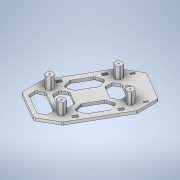
# Autodesk Inventor part: top_body
Saved by Autodesk Inventor 2022 (Build 260153000, 153)
## iProperties
Created: 2022-01-21
Part Number: top_body
Material: Generic
Document SubType Name: Modeling
Designer: felix
Density: 1 g/cm^3
Appearance: Default
Author: felix
Autodesk Inventor part; units mm, degrees
ref_plane "YZ Plane" through (0, 0, 0) normal (1, 0, 0) x (0, 1, 0)
ref_plane "XZ Plane" through (0, 0, 0) normal (0, 1, 0) x (-1, 0, 0)
ref_plane "XY Plane" through (0, 0, 0) normal (0, 0, 1) x (1, 0, 0)
sketch "Sketch1" plane through (0, 0, 0) normal (0, 1, 0) x (-1, 0, 0)
  line L0 (-6.75, 41.2863) -> (6.75, 41.2863)
  line L1 (-8.75, 41.2863) -> (-12.4549, 41.2863)
  line L2 (10.8365, 42.2863) -> (27.4378, 71.0407)
  line L3 (39.1337, 45.1185) -> (-87.6959, 118.3436) construction
  line L4 (27.4378, 73.0407) -> (16.6581, 91.7116)
  line L5 (-8.3003, 49.4105) -> (11.6997, 84.0516) construction
  line L6 (11.6997, 84.0516) -> (-40.2618, 114.0516) construction
  line L7 (-40.2618, 114.0516) -> (-60.2618, 79.4105) construction
  line L8 (-60.2618, 79.4105) -> (-8.3003, 49.4105) construction
  line L9 (27.4378, 73.0407) -> (16.6581, 91.7116)
  line L10 (-13.4549, 41.5543) -> (-38.9716, 56.2863)
  line L11 (15.9261, 92.4437) -> (-9.5906, 107.1757)
  line L12 (-38.9716, 56.2863) -> (-9.5906, 107.1757) construction
  line L13 (8.75, 41.2863) -> (9.1045, 41.2863)
  line L14 (6.75, 41.2863) -> (8.75, 41.2863)
  line L15 (-6.75, 41.2863) -> (-8.75, 41.2863)
  line L16 (-68.0728, 76.691) -> (-74.8228, 88.3824)
  line L17 (-67.0728, 74.959) -> (-65.2203, 71.7504)
  line L18 (-76, 92.4214) -> (-59.4085, 121.1588)
  line L19 (-57.678, 122.1588) -> (-36.1088, 122.1757)
  line L20 (-57.678, 122.1588) -> (-36.1088, 122.1757)
  line L21 (-64.4882, 71.0184) -> (-38.9716, 56.2863)
  line L22 (-35.1072, 121.9078) -> (-9.5906, 107.1757)
  line L23 (-75.8228, 90.1144) -> (-76, 90.4214)
  line L24 (-74.8228, 88.3824) -> (-75.8228, 90.1144)
  line L25 (-68.0728, 76.691) -> (-67.0728, 74.959)
  line L26 (-41.8469, 122.123) -> (-39.8469, 122.123)
  line L27 (8.3465, 47.7755) -> (2.3722, 47.4278)
  line L28 (0.4688, 48.5268) -> (-2.2172, 53.8745)
  line L29 (-2.162, 55.7721) -> (9.2595, 75.5549)
  line L30 (10.8754, 76.5515) -> (16.8496, 76.8992)
  line L31 (18.753, 75.8002) -> (21.439, 70.4525)
  line L32 (21.3839, 68.5549) -> (9.9623, 48.7721)
  line L33 (-53.2912, 79.9841) -> (-55.0232, 76.9841)
  line L34 (-55.4562, 76.7341) -> (-58.9203, 76.7341)
  line L35 (-59.3533, 76.9841) -> (-61.0854, 79.9841)
  line L36 (-61.0854, 80.4841) -> (-59.3533, 83.4841)
  line L37 (-58.9203, 83.7341) -> (-55.4562, 83.7341)
  line L38 (-55.0232, 83.4841) -> (-53.2912, 80.4841)
  circle A0 centre (-57.1883, 80.2341) radius 0.75
  line L39 (-37.2732, 107.728) -> (-35.5412, 110.728)
  line L40 (-35.5412, 111.228) -> (-37.2732, 114.228)
  line L41 (-37.7062, 114.478) -> (-41.1703, 114.478)
  line L42 (-41.6033, 114.228) -> (-43.3354, 111.228)
  line L43 (-43.3354, 110.728) -> (-41.6033, 107.728)
  line L44 (-41.1703, 107.478) -> (-37.7062, 107.478)
  circle A1 centre (-39.4383, 110.978) radius 0.75
  line L45 (-11.2889, 55.7341) -> (-13.021, 52.7341)
  line L46 (-13.021, 52.2341) -> (-11.2889, 49.2341)
  line L47 (-10.8559, 48.9841) -> (-7.3918, 48.9841)
  line L48 (-6.9588, 49.2341) -> (-5.2268, 52.2341)
  line L49 (-5.2268, 52.7341) -> (-6.9588, 55.7341)
  line L50 (-7.3918, 55.9841) -> (-10.8559, 55.9841)
  circle A2 centre (-9.1239, 52.4841) radius 0.75
  line L51 (10.7912, 86.478) -> (12.5232, 83.478)
  line L52 (6.8941, 86.728) -> (10.3582, 86.728)
  line L53 (4.729, 83.478) -> (6.4611, 86.478)
  circle A3 centre (8.6261, 83.228) radius 0.75
  line L54 (12.5232, 82.978) -> (10.7912, 79.978)
  line L55 (10.3582, 79.728) -> (6.8941, 79.728)
  line L56 (6.4611, 79.978) -> (4.729, 82.978)
  line L57 (-55.4676, 69.7144) -> (-53.9676, 72.3125)
  line L58 (-53.9676, 72.3125) -> (-49.6375, 69.8125)
  line L59 (-49.6375, 69.8125) -> (-51.1375, 67.2144)
  line L60 (-51.1375, 67.2144) -> (-55.4676, 69.7144)
  line L61 (-29.4676, 114.7477) -> (-30.9676, 112.1496)
  line L62 (-30.9676, 112.1496) -> (-26.6375, 109.6496)
  line L63 (-26.6375, 109.6496) -> (-25.1375, 112.2477)
  line L64 (-25.1375, 112.2477) -> (-29.4676, 114.7477)
  line L65 (-19.0945, 48.7144) -> (-17.5945, 51.3125)
  line L66 (-17.5945, 51.3125) -> (-21.9247, 53.8125)
  line L67 (-21.9247, 53.8125) -> (-23.4247, 51.2144)
  line L68 (-23.4247, 51.2144) -> (-19.0945, 48.7144)
  line L69 (2.5753, 96.2477) -> (6.9055, 93.7477)
  line L70 (1.0753, 93.6496) -> (2.5753, 96.2477)
  line L71 (5.4055, 91.1496) -> (1.0753, 93.6496)
  line L72 (6.9055, 93.7477) -> (5.4055, 91.1496)
  line L73 (-46.6764, 74.1128) -> (-44.8462, 67.2827)
  line L74 (-43.9144, 66.0683) -> (-28.0288, 56.8967)
  line L75 (-26.5111, 56.6969) -> (-19.681, 58.527)
  line L76 (-18.2668, 60.9765) -> (-20.0969, 67.8067)
  line L77 (-21.0288, 69.0211) -> (-36.9144, 78.1926)
  line L78 (-38.432, 78.3924) -> (-45.2622, 76.5623)
  line L79 (18.1627, 76.9756) -> (1.0591, 47.3514) construction
  line L80 (-47.6318, 61.2863) -> (-30.8691, 90.3203) construction
  line L81 (-30.3113, 51.2863) -> (-13.5486, 80.3203) construction
  line L82 (12.8862, 45.8364) -> (-2.7013, 54.8382) construction
  line L83 (25.3698, 67.436) -> (9.8846, 76.3787) construction
  line L84 (-28.8812, 104.9351) -> (-22.051, 106.7652)
  line L85 (-20.5334, 106.5654) -> (-4.6478, 97.3938)
  line L86 (-3.7159, 96.1794) -> (-1.8858, 89.3493)
  line L87 (-3.3, 86.8998) -> (-10.1301, 85.0696)
  line L88 (-11.6478, 85.2695) -> (-27.5334, 94.441)
  line L89 (-28.4652, 95.6554) -> (-30.2954, 102.4856)
  line L90 (-18.2508, 112.1757) -> (-35.0136, 83.1418) construction
  line L91 (-0.9303, 102.1757) -> (-17.6931, 73.1418) construction
  line L92 (-57.1883, 80.2341) -> (8.6261, 83.228) construction
  line L93 (-9.1239, 52.4841) -> (-39.4383, 110.978) construction
  line L94 (-17.7491, 59.0447) -> (-47.194, 76.0447) construction
  line L95 (-1.3681, 87.4174) -> (-30.813, 104.4174) construction
  line L96 (-52.6468, 88.8704) -> (-40.5224, 81.8704) construction
  line L97 (-44.6468, 102.7268) -> (-32.5224, 95.7268) construction
  line L98 (-36.6156, 102.6371) -> (-48.5536, 81.9601) construction
  line L99 (3.4998, 73.5788) -> (-3.3306, 61.7482)
  line L100 (-5.0849, 60.7484) -> (-10.8215, 60.8124)
  line L101 (-12.5199, 61.793) -> (-15.4436, 66.729)
  line L102 (-15.4549, 68.7482) -> (-8.6245, 80.5788)
  line L103 (-6.8702, 81.5786) -> (-1.1336, 81.5146)
  line L104 (0.5648, 80.534) -> (3.4885, 75.598)
  line L105 (-3.9154, 60.7353) -> (-16.0397, 67.7353) construction
  line L106 (4.0846, 74.5917) -> (-8.0397, 81.5917) construction
  line L107 (-0.0086, 81.502) -> (-11.9465, 60.825) construction
  arc A4 (-57.678, 122.1588) -> (-59.4085, 121.1588) centre (-57.6764, 120.1588) ccw
  arc A5 (-76, 92.4214) -> (-76, 90.4214) centre (-74.2679, 91.4214) ccw
  arc A6 (-35.1072, 121.9078) -> (-36.1088, 122.1757) centre (-36.1072, 120.1757) ccw
  arc A7 (16.6581, 91.7116) -> (15.9261, 92.4437) centre (14.9261, 90.7116) ccw
  arc A8 (27.4378, 71.0407) -> (27.4378, 73.0407) centre (25.7058, 72.0407) ccw
  arc A9 (9.1045, 41.2863) -> (10.8365, 42.2863) centre (9.1045, 43.2863) ccw
  arc A10 (-13.4549, 41.5543) -> (-12.4549, 41.2863) centre (-12.4549, 43.2863) ccw
  arc A11 (-65.2203, 71.7504) -> (-64.4882, 71.0184) centre (-63.4882, 72.7504) ccw
  arc A12 (-61.0854, 80.4841) -> (-61.0854, 79.9841) centre (-60.6524, 80.2341) ccw
  arc A13 (-58.9203, 83.7341) -> (-59.3533, 83.4841) centre (-58.9203, 83.2341) ccw
  arc A14 (-55.0232, 83.4841) -> (-55.4562, 83.7341) centre (-55.4562, 83.2341) ccw
  arc A15 (-53.2912, 79.9841) -> (-53.2912, 80.4841) centre (-53.7242, 80.2341) ccw
  arc A16 (-55.4562, 76.7341) -> (-55.0232, 76.9841) centre (-55.4562, 77.2341) ccw
  arc A17 (-59.3533, 76.9841) -> (-58.9203, 76.7341) centre (-58.9203, 77.2341) ccw
  arc A18 (-43.3354, 111.228) -> (-43.3354, 110.728) centre (-42.9024, 110.978) ccw
  arc A19 (-41.1703, 114.478) -> (-41.6033, 114.228) centre (-41.1703, 113.978) ccw
  arc A20 (-37.2732, 114.228) -> (-37.7062, 114.478) centre (-37.7062, 113.978) ccw
  arc A21 (-35.5412, 110.728) -> (-35.5412, 111.228) centre (-35.9742, 110.978) ccw
  arc A22 (-37.7062, 107.478) -> (-37.2732, 107.728) centre (-37.7062, 107.978) ccw
  arc A23 (-41.6033, 107.728) -> (-41.1703, 107.478) centre (-41.1703, 107.978) ccw
  arc A24 (6.8941, 86.728) -> (6.4611, 86.478) centre (6.8941, 86.228) ccw
  arc A25 (10.7912, 86.478) -> (10.3582, 86.728) centre (10.3582, 86.228) ccw
  arc A26 (12.5232, 82.978) -> (12.5232, 83.478) centre (12.0902, 83.228) ccw
  arc A27 (10.3582, 79.728) -> (10.7912, 79.978) centre (10.3582, 80.228) ccw
  arc A28 (6.4611, 79.978) -> (6.8941, 79.728) centre (6.8941, 80.228) ccw
  arc A29 (4.729, 83.478) -> (4.729, 82.978) centre (5.162, 83.228) ccw
  arc A30 (-13.021, 52.7341) -> (-13.021, 52.2341) centre (-12.588, 52.4841) ccw
  arc A31 (-11.2889, 49.2341) -> (-10.8559, 48.9841) centre (-10.8559, 49.4841) ccw
  arc A32 (-7.3918, 48.9841) -> (-6.9588, 49.2341) centre (-7.3918, 49.4841) ccw
  arc A33 (-5.2268, 52.2341) -> (-5.2268, 52.7341) centre (-5.6598, 52.4841) ccw
  arc A34 (-6.9588, 55.7341) -> (-7.3918, 55.9841) centre (-7.3918, 55.4841) ccw
  arc A35 (-10.8559, 55.9841) -> (-11.2889, 55.7341) centre (-10.8559, 55.4841) ccw
  arc A36 (-45.2622, 76.5623) -> (-46.6764, 74.1128) centre (-44.7445, 74.6305) ccw
  arc A37 (-36.9144, 78.1926) -> (-38.432, 78.3924) centre (-37.9144, 76.4606) ccw
  arc A38 (-44.8462, 67.2827) -> (-43.9144, 66.0683) centre (-42.9144, 67.8003) ccw
  arc A39 (-28.0288, 56.8967) -> (-26.5111, 56.6969) centre (-27.0288, 58.6288) ccw
  arc A40 (-19.681, 58.527) -> (-18.2668, 60.9765) centre (-20.1986, 60.4589) ccw
  arc A41 (-20.0969, 67.8067) -> (-21.0288, 69.0211) centre (-22.0288, 67.289) ccw
  arc A42 (-28.4652, 95.6554) -> (-27.5334, 94.441) centre (-26.5334, 96.1731) ccw
  arc A43 (-28.8812, 104.9351) -> (-30.2954, 102.4856) centre (-28.3635, 103.0032) ccw
  arc A44 (-20.5334, 106.5654) -> (-22.051, 106.7652) centre (-21.5334, 104.8333) ccw
  arc A45 (-3.7159, 96.1794) -> (-4.6478, 97.3938) centre (-5.6478, 95.6618) ccw
  arc A46 (-3.3, 86.8998) -> (-1.8858, 89.3493) centre (-3.8176, 88.8316) ccw
  arc A47 (-11.6478, 85.2695) -> (-10.1301, 85.0696) centre (-10.6478, 87.0015) ccw
  arc A48 (-2.162, 55.7721) -> (-2.2172, 53.8745) centre (-0.43, 54.7721) ccw
  arc A49 (10.8754, 76.5515) -> (9.2595, 75.5549) centre (10.9916, 74.5549) ccw
  arc A50 (18.753, 75.8002) -> (16.8496, 76.8992) centre (16.9658, 74.9026) ccw
  arc A51 (21.3839, 68.5549) -> (21.439, 70.4525) centre (19.6518, 69.5549) ccw
  arc A52 (8.3465, 47.7755) -> (9.9623, 48.7721) centre (8.2303, 49.7721) ccw
  arc A53 (0.4688, 48.5268) -> (2.3722, 47.4278) centre (2.256, 49.4244) ccw
  arc A54 (-15.4549, 68.7482) -> (-15.4436, 66.729) centre (-13.7229, 67.7482) ccw
  arc A55 (-6.8702, 81.5786) -> (-8.6245, 80.5788) centre (-6.8925, 79.5788) ccw
  arc A56 (0.5648, 80.534) -> (-1.1336, 81.5146) centre (-1.156, 79.5147) ccw
  arc A57 (3.4998, 73.5788) -> (3.4885, 75.598) centre (1.7678, 74.5788) ccw
  arc A58 (-5.0849, 60.7484) -> (-3.3306, 61.7482) centre (-5.0626, 62.7482) ccw
  arc A59 (-12.5199, 61.793) -> (-10.8215, 60.8124) centre (-10.7991, 62.8123) ccw
  line L108 (-45.2316, 101.7139) -> (-52.062, 89.8833)
  line L109 (-52.0507, 87.864) -> (-49.127, 82.9281)
  line L110 (-47.4285, 81.9475) -> (-41.692, 81.8834)
  line L111 (-37.7407, 102.6497) -> (-43.4772, 102.7137)
  line L112 (-33.1185, 96.7331) -> (-36.0422, 101.6691)
  line L113 (-39.9376, 82.8833) -> (-33.1072, 94.7139)
  arc A60 (-41.692, 81.8834) -> (-39.9376, 82.8833) centre (-41.6697, 83.8833) ccw
  arc A61 (-33.1072, 94.7139) -> (-33.1185, 96.7331) centre (-34.8393, 95.7139) ccw
  arc A62 (-36.0422, 101.6691) -> (-37.7407, 102.6497) centre (-37.763, 100.6498) ccw
  arc A63 (-43.4772, 102.7137) -> (-45.2316, 101.7139) centre (-43.4995, 100.7139) ccw
  arc A64 (-52.062, 89.8833) -> (-52.0507, 87.864) centre (-50.3299, 88.8833) ccw
  arc A65 (-49.127, 82.9281) -> (-47.4285, 81.9475) centre (-47.4062, 83.9474) ccw
  point P0 (10.2592, 41.2863)
  point P1 (-12.9908, 41.2863)
  point P2 (28.0152, 72.0407)
  point P3 (19.1372, 56.6635)
  point P4 (-67.6993, 106.7986)
  point P5 (-8.3003, 49.4105)
  point P6 (-24.2811, 81.731)
  point P7 (9.4231, 47.8382)
  point P8 (21.9231, 69.4888)
  point P9 (-53.1468, 80.2341)
  point P10 (-55.1676, 76.7341)
  point P11 (-59.209, 76.7341)
  point P12 (-61.2297, 80.2341)
  point P13 (-59.209, 83.7341)
  point P14 (-55.1676, 83.7341)
  point P15 (-37.4176, 107.478)
  point P16 (-35.3968, 110.978)
  point P17 (-37.4176, 114.478)
  point P18 (-41.459, 114.478)
  point P19 (-43.4797, 110.978)
  point P20 (-41.459, 107.478)
  point P21 (-11.1446, 55.9841)
  point P22 (-13.1653, 52.4841)
  point P23 (-11.1446, 48.9841)
  point P24 (-7.1031, 48.9841)
  point P25 (-5.0824, 52.4841)
  point P26 (-7.1031, 55.9841)
  point P27 (10.6469, 86.728)
  point P28 (12.6676, 83.228)
  point P29 (6.6054, 86.728)
  point P30 (4.5847, 83.228)
  point P31 (10.6469, 79.728)
  point P32 (6.6054, 79.728)
  point P33 (-44.6318, 66.4825)
  point P34 (-27.3113, 56.4825)
  point P35 (-20.3113, 68.6069)
  point P36 (-37.6318, 78.6069)
  point P37 (-21.2508, 106.9796)
  point P38 (-3.9303, 96.9796)
  point P39 (-10.9303, 84.8552)
  point P40 (-28.2508, 94.8552)
  point P41 (8.6261, 83.228)
  dimension "d82" = 23.25
  dimension "d88" = 120
  dimension "d89" = 120
  dimension "d90" = 35.512
  dimension "d91" = 17.756
  dimension "d92" = 17.756
  dimension "d95" = 40
  dimension "d97" = 20
  dimension "d99" = 30
  dimension "d102" = 60
  dimension "d145" = 180
  dimension "d146" = 30
  dimension "d147" = 8.1242
  dimension "d148" = 8.1242
  dimension "d155" = 1.5
  dimension "d156" = 7
  dimension "d157" = 1.5
  dimension "d158" = 1.5
  dimension "d160" = 3
  dimension "d162" = 3
  dimension "d163" = 9
  dimension "d169" = 6
  dimension "d170" = 10
  dimension "d171" = 20
  dimension "d172" = 14
  dimension "d179" = 7
  dimension "d181" = 2
  dimension "d186" = 0.5
  dimension "d187" = 0.5
  dimension "d189" = 2
  dimension "d190" = 2
  dimension "d191" = 4
  dimension "d192" = 16
  dimension "d193" = 8
  dimension "d194" = 14
  dimension "d195" = 8
  dimension "d204" = 14
  dimension "d206" = 18.762
  dimension "d207" = 28.2702
  dimension "d238" = 5
  dimension "d244" = 25
  dimension "d245" = 12.5
  dimension "d246" = 0
  dimension "d247" = 4
  constraints: 228 end point, 124 point on circle, 112 tangent, 105 point on line, 79 symmetric about line, 66 centre point, 51 equal radius, 16 parallel, 9 equal length, 6 perpendicular, 4 collinear, 3 coincident, 3 midpoint, 2 horizontal, 27 other
  measures "d82" distance of point (10.259, 41.286) point (-12.991, 41.286)
  measures "d88" angle of L2 L1
  measures "d89" angle of L4 L2
  measures "d90" distance of point (10.259, 41.286) point (28.015, 72.041)
  measures "d91" distance of point (19.137, 56.663) point (10.259, 41.286)
  measures "d92" distance of point (28.015, 72.041) point (19.137, 56.663)
  measures "d95" distance of L5.start L5.end
  measures "d97" distance from line of L3 L5.start
  measures "d99" distance of L10.end point (-12.991, 41.286)
  measures "d102" distance of L7.end L5.start
  measures "d145" angle of L10 L21
  measures "d146" distance from line of L5 point (-24.281, 81.731)
  measures "d147" distance from line of L0 L5.start
  measures "d148" distance from line of L4 L5.end
  measures "d155" diameter of A0
  measures "d156" distance between parallel lines of L38 L35
  measures "d157" distance edge to line of A0 L7
  measures "d158" distance edge to line of A0 L8
  measures "d160" distance between parallel lines of L58 L60
  measures "d162" distance between parallel lines of L8 L58
  measures "d163" distance between parallel lines of L57 L7
  measures "d169" distance between parallel lines of L21 L74
  measures "d170" distance from line of L12 point (-27.311, 56.482)
  measures "d171" distance of point (-44.632, 66.482) point (-27.311, 56.482)
  measures "d172" distance between parallel lines of L77 L74
  measures "d179" distance from line of L94.end L80
  measures "d181" radius of A4
  measures "d186" radius of A12
  measures "d187" radius of A27
  measures "d189" radius of A36
  measures "d190" radius of A54
  measures "d191" distance between parallel lines of L29 L99
  measures "d192" distance of L105.start L106.start
  measures "d193" distance from line of L3 L106.start
  measures "d194" distance between parallel lines of L99 L102
  measures "d195" distance between parallel lines of L106 L3
  measures "d204" distance between parallel lines of L32 L29
  measures "d206" distance between parallel lines of L88 L77
  measures "d207" distance between parallel lines of L113 L102
  measures "d238" distance of L59.end L57.start
  measures "d244" distance of point (21.923, 69.489) point (9.423, 47.838)
  measures "d245" distance from line of L3 point (9.423, 47.838)
  measures "d246" angle of L83 L82
  measures "d247" distance between parallel lines of L2 L32
extrude "Extrusion1_main_body" add sketch "Sketch1" along normal blind 3 contours L15 L1 A10 L10 L21 A11 L17 L25 L16 L24 L23 A5 L18 A4 L19 A6 L22 L11 A7 L4 A8 L2 A9 L13 L14 L0
extrude "Extrusion2_main_body" add sketch "Sketch1" along normal blind 16 contours L33 A16 L34 A17 L35 A12 L36 A13 L37 A14 L38 A15 | A22 L44 A23 L43 A18 L42 A19 L41 A20 L40 A21 L39 | A35 L50 A34 L49 A33 L48 A32 L47 A31 L46 A30 L45 | L51 A26 L54 A27 L55 A28 L56 A29 L53 A24 L52 A25
extrude "Extrusion3_main_body" add sketch "Sketch1" along normal blind 13 contours A0 | A1 | A2 | A3
sketch "Sketch2_insert" plane through (0, 0, 0) normal (0, -1, 0) x (1, 0, 0)
  line L0 (43.2139, 119.2087) -> (66.2139, 79.3715)
  line L1 (66.2139, 79.3715) -> (65.0014, 78.6715)
  line L2 (65.0014, 78.6715) -> (42.0014, 118.5087)
  line L3 (42.0014, 118.5087) -> (43.2139, 119.2087)
  line L4 (59.4085, 121.1588) -> (76, 92.4214) projected
  line L5 (52.062, 89.8833) -> (45.2316, 101.7139) projected
  line L6 (64.4882, 71.0184) -> (13.4549, 41.5543) projected
  line L7 (-15.9261, 92.4437) -> (35.1072, 121.9078) projected
  line L8 (66.7315, 106.2285) -> (52.402, 97.9553) construction
  line L9 (59.4085, 121.1588) -> (76, 92.4214) projected
  line L10 (51.0014, 102.9202) -> (47.5373, 100.9202)
  line L11 (47.5373, 100.9202) -> (52.5373, 92.26)
  line L12 (52.5373, 92.26) -> (56.0014, 94.26)
  line L13 (52.2139, 103.6202) -> (53.9459, 104.6202)
  line L14 (53.9459, 104.6202) -> (58.9459, 95.96)
  line L15 (58.9459, 95.96) -> (57.2139, 94.96)
  line L16 (46.5289, 118.4668) -> (49.993, 120.4668)
  line L17 (49.993, 120.4668) -> (50.993, 118.7348)
  line L18 (50.993, 118.7348) -> (47.5289, 116.7348)
  line L19 (47.5289, 116.7348) -> (46.5289, 118.4668)
  line L20 (36.1088, 122.1757) -> (57.678, 122.1588) projected
  line L21 (67.2289, 82.6134) -> (70.693, 84.6134)
  line L22 (70.693, 84.6134) -> (69.693, 86.3454)
  line L23 (69.693, 86.3454) -> (66.2289, 84.3454)
  line L24 (66.2289, 84.3454) -> (67.2289, 82.6134)
  point P0 (0, 0)
  point P1 (54.7139, 99.2901)
  point P2 (67.7042, 106.7901)
  point P3 (50.0373, 96.5901)
  dimension "d249" = 1.4
  dimension "d250" = 15
  dimension "d251" = 46
  dimension "d252" = 23
  dimension "d254" = 10
  dimension "d255" = 4
  dimension "d256" = 1.6
  dimension "d257" = 10
  dimension "d258" = 2
  dimension "d265" = 4
  dimension "d266" = 2
  dimension "d267" = 2.5
  dimension "d268" = 2.3
  dimension "d269" = 1.698
  constraints: 38 end point, 12 parallel, 7 point on line, 6 perpendicular, 4 symmetric about line, 3 midpoint
  measures "d249" distance of L2.end L0.start
  measures "d250" distance between parallel lines of L4 L0
  measures "d251" distance of L0.start L0.end
  measures "d252" distance of L0.start point (54.714, 99.29)
  measures "d254" distance between parallel lines of L12 L10
  measures "d255" distance of L11.end L12.end
  measures "d256" distance between parallel lines of L5 L11
  measures "d257" distance of L13.end L14.end
  measures "d258" distance of L13.start L13.end
  measures "d265" distance of L16.start L16.end
  measures "d266" distance between parallel lines of L18 L16
  measures "d267" distance between parallel lines of L0 L19
  measures "d268" distance between parallel lines of L16 L3
  measures "d269" distance from line of L16.end L20
extrude "Extrusion1_feature1" cut sketch "Sketch2_insert" against normal blind 1.5 contours L0 L1 L2 L3
extrude "Extrusion2_feature1" cut sketch "Sketch2_insert" against normal blind 1.2 contours L13 L14 L15 L0
extrude "Extrusion3_feature1" cut sketch "Sketch2_insert" against normal blind 3 contours L2 L12 L11 L10
extrude "Extrusion4_feature1_zip_ties" cut sketch "Sketch2_insert" against normal blind 3 contours L16 L17 L18 L19 | L24 L23 L22 L21
body "Solid1"
